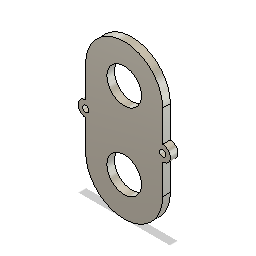
Shooter+motor+gard (Autodesk Fusion 360 design; units mm, degrees)
Autodesk Fusion 360 part; units mm, degrees
sketch "Sketch1" plane through (0, 0, 0) normal (0, 0, 1) x (1, 0, 0)
  arc A0 (31.75, 63.5) -> (-31.75, 63.5) centre (0, 63.5) ccw
  arc A1 (-31.75, 0) -> (31.75, 0) centre (0, 0) ccw
  line L0 (0, 0) -> (0, 63.5) construction
  circle A2 centre (0, 63.5) radius 14.2748
  circle A3 centre (0, 0) radius 14.2748
  arc A4 (-31.75, 37.5429) -> (-31.75, 24.8429) centre (-31.75, 31.1929) ccw
  arc A5 (31.75, 24.8429) -> (31.75, 37.5429) centre (31.75, 31.1929) ccw
  line L1 (-31.75, 63.5) -> (-31.75, 37.5429)
  line L2 (-31.75, 24.8429) -> (-31.75, 0)
  line L3 (31.75, 0) -> (31.75, 24.8429)
  line L4 (31.75, 37.5429) -> (31.75, 63.5)
  circle A6 centre (0, 0) radius 31.75 construction
  circle A7 centre (0, 63.5) radius 31.75 construction
  circle A8 centre (31.75, 31.1929) radius 2.5797
  circle A9 centre (-31.75, 31.1929) radius 2.5797
  dimension "d1" = 63.5
  dimension "d2" = 28.5496
  dimension "d3" = 28.5496
  dimension "d4" = 63.5
  dimension "d5" = 12.7
  dimension "d6" = 12.7
  dimension "d7" = 63.5
  dimension "d8" = 63.5
  dimension "d9" = 5.1594
  dimension "d10" = 5.1594
  constraint tangent A0 L3
  constraint tangent A0 L1
  constraint parallel L1 L3
  constraint tangent A1 L1
  constraint tangent A1 L3
  constraint vertical L0
  constraint coincident A1.centre L0.start
  constraint concentric A0 A2
  constraint concentric A1 A3
  constraint coincident A4.end L1
  constraint coincident A5.end L3
  constraint collinear L1 L2
  constraint coincident A4.centre L1
  constraint collinear L3 L4
  constraint coincident A5.centre L3
  constraint concentric A0 A7
  constraint concentric A5 A8
  constraint concentric A4 A9
  measures "d1" diameter of A0
  measures "d2" diameter of A2
  measures "d3" diameter of A3
  measures "d4" distance of A0.centre A1.centre
  measures "d5" diameter of A4
  measures "d6" diameter of A5
  measures "d7" diameter of A6
  measures "d8" diameter of A7
  measures "d9" diameter of A8
  measures "d10" diameter of A9
extrude "Extrude1" add sketch "Sketch1" along normal blind 6.35
equation "d9 = ( 13 / 64 ) * 1 in"
equation "d10 = ( 13 / 64 ) * 1 in"
